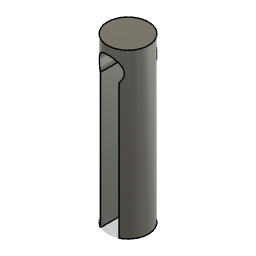
key_hole (Autodesk Fusion 360 design; units mm, degrees)
Autodesk Fusion 360 part; units mm, degrees
sketch "Sketch1" plane through (0, 0, 0) normal (0, 1, 0) x (1, 0, 0)
  circle A0 centre (0, 0) radius 5
  constraint coincident A0.centre origin
extrude "Extrude1" add sketch "Sketch1" against normal blind 35
extrude "Extrude2" add 1 faces at (1.3101, 0, 1.9935) along direction (0, 1, 0) blind 5
ref_plane "WorkPlane1" through (0, -1.4815, 5) normal (0, 0, 1) x (1, 0, 0)
sketch "Sketch2" plane through (0, 0, 5) normal (0, 0, 1) x (1, 0, 0)
  circle A0 centre (0, 0) radius 3.05
  line L0 (0, 0) -> (-2.25, 0)
  line L1 (-2.25, 0) -> (-2.25, -35)
  line L2 (-2.25, -35) -> (0, -35)
  line L3 (0, -35) -> (0, 0)
  line L4 (0, 0) -> (2.25, 0)
  line L5 (2.25, 0) -> (2.25, -35)
  line L6 (2.25, -35) -> (0, -35)
  line L7 (0, -35) -> (0, 0)
  constraint coincident A0.centre L0.start
  constraint horizontal L0
  constraint vertical L1
  constraint horizontal L2
  constraint vertical L3
  constraint horizontal L4
  constraint vertical L5
  constraint horizontal L6
  constraint vertical L7
  constraint equal L2 L6
extrude "Extrude3" cut sketch "Sketch2" against normal blind 16
equation "d7 = 2 * 3.05 mm"
